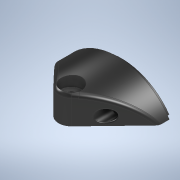
# Autodesk Inventor part: WheelBracketHead_V4
Saved by Autodesk Inventor 2020 (Build 240168000, 168)
## iProperties
Created: 2020-01-04
Part Number: WheelBracketHead_V4
Material: ABS Plastic
Document SubType Name: Modeling
Designer: Connor
Density: 1.06 g/cm^3
Appearance: Glossy - Black
Author: Connor
Autodesk Inventor part; units mm, degrees
ref_plane "YZ Plane" through (0, 0, 0) normal (1, 0, 0) x (0, 1, 0)
ref_plane "XZ Plane" through (0, 0, 0) normal (0, 1, 0) x (-1, 0, 0)
ref_plane "XY Plane" through (0, 0, 0) normal (0, 0, 1) x (1, 0, 0)
sketch "Sketch1" plane through (0, 0, 0) normal (0, 1, 0) x (-1, 0, 0)
  line L0 (0, 0) -> (-46.99, 0)
  line L1 (-46.99, 0) -> (-46.99, -44.45)
  line L2 (-46.99, -44.45) -> (0, -44.45)
  line L3 (0, -44.45) -> (0, 0)
  line L4 (0, -44.45) -> (46.99, -44.45)
  line L5 (46.99, -44.45) -> (46.99, 0)
  line L6 (46.99, 0) -> (0, 0)
  line L7 (0, -44.45) -> (0, -47.625)
  line L8 (0, -47.625) -> (-44.196, -47.625)
  line L9 (-44.196, -47.625) -> (-44.196, -44.45)
  circle A0 centre (0, -9.525) radius 3.175
  circle A1 centre (0, -9.525) radius 9.525
  line L10 (46.99, -44.45) -> (6.8499, -2.9065)
  line L11 (-46.99, -44.45) -> (-6.8499, -2.9065)
  line L12 (0, -47.625) -> (44.196, -47.625)
  line L13 (44.196, -47.625) -> (44.196, -44.45)
  dimension "d0" = 46.99
  dimension "d1" = 3.175
  dimension "d2" = 44.196
  dimension "d3" = 6.35
  dimension "d4" = 6.35
  dimension "d5" = 34.925
  constraints: 28 end point, 5 perpendicular, 4 horizontal, 3 point on line, 3 tangent, 2 centre point, 2 collinear, 2 parallel, 2 point on circle, 1 vertical
  measures "d0" distance of L1.end L2.end
  measures "d1" distance of L8.end L9.end
  measures "d2" distance of L7.end L8.end
  measures "d3" diameter of A0
  measures "d4" radial gap between concentric circles of A0 A1
  measures "d5" distance from line of A0.centre L4
revolve "Revolution1" add sketch "Sketch1" angle 180 about axis through (0, 0, -44.45) along (0, 0, 1) picked at (-0.7359, -16.8469) picked at (-0.4918, -10.4621) contours A1 L11 L1 L0 | L3 A0 A1 | L3 A0 | A1 L3 L2 L11 | L2 L7 L8 L9
extrude "Extrusion1" cut sketch "Sketch1" along normal blind 25.4
extrude "Extrusion2" cut sketch "Sketch1" along normal through all contours A1 L11 L1 L0 | L6 L5 L10 A1
sketch "Sketch2" plane through (0, 0, 0) normal (0, 0, 1) x (1, 0, 0)
  circle A0 centre (0, 0) radius 37.0265 construction
  point P0 (-19.05, 31.75)
  point P1 (19.05, 31.75)
  dimension "d11" = 38.1
  dimension "d12" = 31.75
  constraints: 2 point on circle, 1 centre point, 1 coincident, 1 horizontal alignment
  measures "d11" distance of A0.end A0.start
  measures "d12" vertical distance of point (0, 0) A0.end
hole "Hole1" at (-19.05, 31.75, 0) at (19.05, 31.75, 0) direction (0, 0, -1) diameter 5.207 end through all counterbore diameter 8.7313 counterbore depth 25.4
ref_plane "Work Plane1" through (0, 46.99, -22.225) normal (0, -1, 0) x (1, 0, 0)
sketch "Sketch3" plane through (0, 46.99, -22.225) normal (0, -1, 0) x (1, 0, 0)
  arc A0 (6.8499, 19.3185) -> (-6.8499, 19.3185) centre (0, 12.7) ccw projected
  point P0 (0, 22.225)
  constraints: 1 coincident
hole "Hole2" at (0, 46.99, -9.525) direction (0, -1, 0) diameter 6.7564 end through all counterbore diameter 15.875 counterbore depth 7.9502
sketch "Sketch5" plane through (0, 0, -47.625) normal (0, 0, -1) x (-1, 0, 0)
  circle A0 centre (0, 0) radius 41.275
  line L0 (12.7, 39.2726) -> (12.7, -39.2726)
  line L1 (-12.7, 39.2726) -> (-12.7, -39.2726)
  dimension "d30" = 82.55
  dimension "d31" = 25.4
  constraints: 4 end point, 4 point on circle, 2 vertical, 1 centre point, 1 coincident, 1 parallel
  measures "d30" diameter of A0
  measures "d31" distance between parallel lines of L1 L0
extrude "Extrusion4" cut sketch "Sketch5" against normal blind 12.7 contours L0 A0 L1
sketch "Sketch8" plane through (0, 0, 0) normal (1, 0, 0) x (0, 1, 0)
  line L0 (30.48, -34.925) -> (30.48, -22.225)
  line L1 (30.48, -22.225) -> (20.9585, -22.225)
  line L2 (20.9585, -22.225) -> (16.1925, -30.48)
  line L3 (16.1925, -34.925) -> (30.48, -34.925)
  line L4 (25.4, -12.9032) -> (25.4, -6.1468) projected
  line L5 (16.1925, -30.48) -> (16.1925, -34.925)
  line L6 (25.4, -34.925) -> (39.2726, -34.925) projected
  point P0 (0, 0)
  point P1 (25.4, -9.525)
  dimension "d45" = 120
  dimension "d49" = 30.48
  dimension "d52" = 8.255
  dimension "d53" = 12.7
  dimension "d54" = 14.2875
  constraints: 10 end point, 2 vertical, 1 collinear, 1 midpoint, 1 parallel, 1 perpendicular
  measures "d45" angle of L2 L1
  measures "d49" distance from line of point (0, 0) L0
  measures "d52" vertical distance of L2.end L1.end
  measures "d53" distance from line of point (25.4, -9.525) L1
  measures "d54" distance of L3.start L0.start
revolve "Revolution2" cut sketch "Sketch8" angle 360 about axis through (0, 30.48, -34.925) along (0, 0, 1)
sketch "Sketch9" plane through (0, 30.48, -22.225) normal (0, 0, -1) x (-1, 0, 0)
  arc A0 (8.0531, -5.08) -> (-8.0531, -5.08) centre (0, 0) ccw projected
  point P0 (0, -30.48)
  constraints: 1 coincident
hole "Hole4" at (0, 30.48, -22.225) direction (0, 0, 1) diameter 8.89 depth 6.35 counterbore diameter 12.954 counterbore depth 4.7752
fillet "Fillet1" radius 3.175 6 edges at (3.9366, 46.8248, -0.8515) (-3.9366, 46.8248, -0.8515) (-25.4761, 39.4845, -22.1839) (25.4761, 39.4845, -22.1839) (-12.7, 39.2726, -41.275) (12.7, 39.2726, -41.275)
fillet "Fillet2" radius 0.7937 2 edges at (19.05, 36.1156, -15.5331) (-19.05, 36.1156, -15.5331)
body "Solid1"
